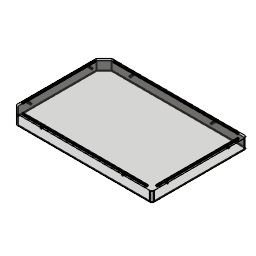
Design_2_Assembly (Autodesk Fusion 360 archive; units mm, degrees)
design "GREINER 96 WELL PLATE LID"
part number: 2026-02-05-10-27-23-618
Autodesk Fusion 360 part; units mm, degrees
sketch "Sketch1" plane through (0, 0, 0) normal (0, 0, 1) x (1, 0, 0)
  line L0 (61.42, -42.3) -> (-56.55, -42.3)
  line L1 (-63.55, -35.3) -> (-63.55, 35.3)
  line L2 (-56.55, 42.3) -> (61.42, 42.3)
  line L3 (63.55, 40.17) -> (63.55, -40.17)
  line L4 (63.55, -42.3) -> (-63.55, 42.3) construction
  line L5 (-63.55, -42.3) -> (63.55, 42.3) construction
  line L6 (-56.55, 42.3) -> (-63.55, 35.3)
  line L7 (0, -42.3) -> (0, 42.3) construction
  line L8 (63.55, 0) -> (-63.55, 0) construction
  line L9 (-56.55, -42.3) -> (-63.55, -35.3)
  arc A0 (63.55, 40.17) -> (61.42, 42.3) centre (61.42, 40.17) ccw
  arc A1 (61.42, -42.3) -> (63.55, -40.17) centre (61.42, -40.17) ccw
  dimension "d1" = 84.6
  dimension "d2" = 127.1
  dimension "d3" = 7
  dimension "d4" = 7
  dimension "d5" = 2.13
  constraint horizontal L0
  constraint perpendicular L0 L1
  constraint parallel L0 L2
  constraint parallel L1 L3
  constraint coincident L4 origin
  constraint coincident L5 origin
  constraint coincident L4.end L2
  constraint coincident L4.end L1
  constraint coincident L2 L7.end
  constraint perpendicular L2 L7
  constraint coincident L1 L8.end
  constraint perpendicular L1 L8
  constraint symmetric L2.start L8 L0.end
  constraint symmetric L1.end L8 L1.start
  constraint coincident L0 L7.start
  constraint coincident L3 L8.start
  constraint coincident L5.end L2
  constraint coincident L5.end L3
  constraint tangent L2 A0
  constraint tangent L3 A0
  constraint symmetric L8 L2.end L0.start
  constraint symmetric L8 L3.start L3.end
  constraint symmetric L8 A0 A1
  measures "d1" distance of L5.start L4.end
  measures "d2" distance of L4.end L5.end
  measures "d3" distance of L4.end L2.start
  measures "d4" distance of L4.end L1.end
  measures "d5" radius of A0
extrude "Extrude1" add sketch "Sketch1" against normal blind 9
sketch "Sketch2" plane through (0, 0, -9) normal (0, 0, -1) x (1, 0, 0)
  line L0 (61.42, 42.3) -> (-56.55, 42.3)
  line L1 (-56.55, 42.3) -> (-63.55, 35.3)
  line L2 (-63.55, 35.3) -> (-63.55, -35.3)
  line L3 (-63.55, -35.3) -> (-56.55, -42.3)
  line L4 (-56.55, -42.3) -> (61.42, -42.3)
  arc A0 (61.42, -42.3) -> (63.55, -40.17) centre (61.42, -40.17) ccw
  line L5 (63.55, -40.17) -> (63.55, 40.17)
  arc A1 (63.55, 40.17) -> (61.42, 42.3) centre (61.42, 40.17) ccw
  line L6 (61.42, -41.3) -> (-56.1358, -41.3)
  line L7 (-62.55, -34.8858) -> (-62.55, 34.8858)
  line L8 (-56.1358, 41.3) -> (61.42, 41.3)
  line L9 (62.55, 40.17) -> (62.55, -40.17)
  line L10 (62.55, -41.3) -> (-62.55, 41.3) construction
  line L11 (-62.55, -41.3) -> (62.55, 41.3) construction
  line L12 (-56.1358, 41.3) -> (-62.55, 34.8858)
  arc A2 (62.55, 40.17) -> (61.42, 41.3) centre (61.42, 40.17) ccw
  line L13 (63.55, 0) -> (-63.55, 0) construction
  line L14 (-56.1358, -41.3) -> (-62.55, -34.8858)
  arc A3 (61.42, -41.3) -> (62.55, -40.17) centre (61.42, -40.17) ccw
  dimension "d8" = 125.1
  dimension "d9" = 82.6
  dimension "d10" = 6.4142
  dimension "d11" = 6.4142
  dimension "d12" = 1
  dimension "d13" = 1.13
  constraint horizontal L6
  constraint perpendicular L6 L7
  constraint parallel L6 L8
  constraint parallel L7 L9
  constraint coincident L10 origin
  constraint coincident L11 origin
  constraint coincident L10.end L8
  constraint coincident L10.end L7
  constraint coincident L11.end L9
  constraint coincident L11.end L8
  constraint tangent L9 A2
  constraint tangent L8 A2
  constraint midpoint L5 L13.start
  constraint midpoint L2 L13.end
  constraint symmetric L8.start L13 L6.end
  constraint symmetric L7.end L13 L7.start
  constraint symmetric L9.start L13 L9.end
  constraint symmetric L8.end L13 L6.start
  constraint symmetric A2 L13 A3
  measures "d8" distance of L10.end L11.end
  measures "d9" distance of L11.start L10.end
  measures "d10" distance of L10.end L8.start
  measures "d11" distance of L10.end L7.end
  measures "d12" distance of L1 L12
  measures "d13" radius of A2
extrude "Extrude2" cut sketch "Sketch2" against normal blind 8 contours L6 L7 L8 L9 L12 A2 L14 A3
sketch "Sketch3" plane through (0, 0, -1) normal (0, 0, -1) x (1, 0, 0)
  line L0 (-56.1358, -41.3) -> (61.42, -41.3)
  arc A0 (61.42, -41.3) -> (62.55, -40.17) centre (61.42, -40.17) ccw
  line L1 (62.55, -40.17) -> (62.55, 40.17)
  arc A1 (62.55, 40.17) -> (61.42, 41.3) centre (61.42, 40.17) ccw
  line L2 (61.42, 41.3) -> (-56.1358, 41.3)
  line L3 (-56.1358, 41.3) -> (-62.55, 34.8858)
  line L4 (-62.55, 34.8858) -> (-62.55, -34.8858)
  line L5 (-62.55, -34.8858) -> (-56.1358, -41.3)
  line L6 (-62.55, 32.8642) -> (-35.55, 32.8642) construction
  line L7 (-35.55, 32.8642) -> (-35.55, 41.3) construction
  line L8 (-35.55, 41.3) -> (-36.55, 41.3)
  line L9 (-36.55, 41.3) -> (-36.55, 37.5)
  line L10 (-36.55, 37.5) -> (-35.55, 37.5)
  line L11 (-35.55, 37.5) -> (-35.55, 41.3)
  line L12 (-50.2731, 41.3) -> (-50.2731, 26.6) construction
  line L13 (-50.2731, 26.6) -> (-62.55, 26.6) construction
  line L14 (-62.55, 26.6) -> (-58.75, 26.6)
  line L15 (-58.75, 26.6) -> (-58.75, 27.6)
  line L16 (-58.75, 27.6) -> (-62.55, 27.6)
  line L17 (-62.55, 27.6) -> (-62.55, 26.6)
  line L18 (62.55, 0) -> (-62.55, 0) construction
  line L19 (-62.55, 30.673) -> (-62.55, 55) construction
  line L20 (62.55, 34.8173) -> (62.55, 55) construction
  line L21 (62.55, 55) -> (-62.55, 55) construction
  line L22 (0, 55) -> (0, -41.3) construction
  line L23 (62.55, 27.6) -> (62.55, 26.6)
  line L24 (62.55, 26.6) -> (58.75, 26.6)
  line L25 (58.75, 27.6) -> (62.55, 27.6)
  line L26 (58.75, 26.6) -> (58.75, 27.6)
  line L27 (36.55, 41.3) -> (36.55, 37.5)
  line L28 (35.55, 37.5) -> (35.55, 41.3)
  line L29 (36.55, 37.5) -> (35.55, 37.5)
  line L30 (35.55, 41.3) -> (36.55, 41.3)
  line L31 (62.55, -26.6) -> (58.75, -26.6)
  line L32 (58.75, -27.6) -> (62.55, -27.6)
  line L33 (58.75, -26.6) -> (58.75, -27.6)
  line L34 (35.55, -37.5) -> (35.55, -41.3)
  line L35 (36.55, -37.5) -> (35.55, -37.5)
  line L36 (36.55, -41.3) -> (36.55, -37.5)
  line L37 (62.55, -27.6) -> (62.55, -26.6)
  line L38 (35.55, -41.3) -> (36.55, -41.3)
  line L39 (-58.75, -26.6) -> (-58.75, -27.6)
  line L40 (-62.55, -26.6) -> (-58.75, -26.6)
  line L41 (-58.75, -27.6) -> (-62.55, -27.6)
  line L42 (-62.55, -27.6) -> (-62.55, -26.6)
  line L43 (-36.55, -37.5) -> (-35.55, -37.5)
  line L44 (-35.55, -37.5) -> (-35.55, -41.3)
  line L45 (-36.55, -41.3) -> (-36.55, -37.5)
  line L46 (-35.55, -41.3) -> (-36.55, -41.3)
  dimension "d16" = 27
  dimension "d17" = 3.8
  dimension "d18" = 1
  dimension "d19" = 14.7
  dimension "d20" = 3.8
  dimension "d21" = 1
  constraint coincident L4 L6.start
  constraint perpendicular L4 L6
  constraint coincident L2 L7.end
  constraint perpendicular L2 L7
  constraint horizontal L8
  constraint vertical L9
  constraint horizontal L10
  constraint vertical L11
  constraint coincident L2 L12.start
  constraint perpendicular L2 L12
  constraint coincident L4 L13.end
  constraint perpendicular L4 L13
  constraint horizontal L14
  constraint vertical L15
  constraint horizontal L16
  constraint vertical L17
  constraint midpoint L1 L18.start
  constraint midpoint L4 L18.end
  constraint coincident L4 L19.start
  constraint perpendicular L6 L19
  constraint coincident L1 L20.start
  constraint parallel L1 L20
  constraint perpendicular L19 L21
  constraint midpoint L21 L22.start
  constraint coincident L0 L22.end
  constraint perpendicular L0 L22
  constraint symmetric L7.end L22 L28.end
  constraint symmetric L8.end L22 L27.start
  constraint symmetric L9.end L22 L27.end
  constraint symmetric L10.end L22 L28.start
  constraint symmetric L13.end L22 L23.end
  constraint symmetric L14.end L22 L24.end
  constraint symmetric L15.end L22 L25.start
  constraint symmetric L16.end L22 L23.start
  constraint symmetric L7.end L18 L44.end
  constraint symmetric L8.end L18 L45.start
  constraint symmetric L9.end L18 L43.start
  constraint symmetric L10.end L18 L43.end
  constraint symmetric L13.end L18 L40.start
  constraint symmetric L14.end L18 L39.start
  constraint symmetric L15.end L18 L39.end
  constraint symmetric L16.end L18 L41.end
  constraint symmetric L18 L23.start L32.end
  constraint symmetric L18 L23.end L31.start
  constraint symmetric L18 L27.end L35.start
  constraint symmetric L18 L28.start L34.start
  constraint symmetric L18 L24.end L31.end
  constraint symmetric L18 L25.start L32.start
  constraint symmetric L18 L27.start L36.start
  constraint symmetric L18 L28.end L34.end
  measures "d16" distance of L6.start L6.end
  measures "d17" distance of L8.end L9.end
  measures "d18" distance of L9.end L10.end
  measures "d19" distance of L12.start L12.end
  measures "d20" distance of L15.end L16.end
  measures "d21" distance of L14.end L15.end
extrude "Extrude3" add sketch "Sketch3" along normal blind 1 contours L0 L43 L44 L45 L46 | L4 L39 L40 L41 L42 | L0 L34 L35 L36 L38 | L4 L14 L15 L16 L17 | L1 L31 L32 L33 L37 | L2 L8 L9 L10 L11 | L1 L23 L24 L25 L26 | L2 L27 L28 L29 L30
sketch "Sketch4" plane through (0, 0, 0) normal (0, 0, 1) x (-1, 0, 0)
  line L0 (56.55, 42.3) -> (-61.42, 42.3)
  arc A0 (-61.42, 42.3) -> (-63.55, 40.17) centre (-61.42, 40.17) ccw
  line L1 (-63.55, 40.17) -> (-63.55, -40.17)
  arc A1 (-63.55, -40.17) -> (-61.42, -42.3) centre (-61.42, -40.17) ccw
  line L2 (-61.42, -42.3) -> (56.55, -42.3)
  line L3 (56.55, -42.3) -> (63.55, -35.3)
  line L4 (63.55, -35.3) -> (63.55, 35.3)
  line L5 (63.55, 35.3) -> (56.55, 42.3)
  line L6 (-63.55, -34.3916) -> (-62.25, -34.3916) construction
  line L7 (-62.25, -34.3916) -> (-62.25, -36.4) construction
  line L8 (-60, -42.3) -> (-66.2, -42.3) construction
  line L9 (-63.55, -39.2433) -> (-63.55, -43.1) construction
  line L10 (-62.25, -36.4) -> (-60.95, -36.4)
  line L11 (-60.95, -36.4) -> (-60.95, 36.4)
  line L12 (-60.95, 36.4) -> (-62.25, 36.4)
  line L13 (-62.25, 36.4) -> (-62.25, -36.4)
  line L14 (-52.6219, -42.3) -> (-52.6219, -41) construction
  line L15 (-52.6219, -41) -> (-57.65, -41) construction
  line L16 (-57.65, -41) -> (53.05, -41)
  line L17 (53.05, -41) -> (53.05, -39.7)
  line L18 (53.05, -39.7) -> (-57.65, -39.7)
  line L19 (-57.65, -39.7) -> (-57.65, -41)
  line L20 (53.05, 39.7) -> (-57.65, 39.7)
  line L21 (-57.65, 41) -> (53.05, 41)
  line L22 (-57.65, 39.7) -> (-57.65, 41)
  line L23 (53.05, 41) -> (53.05, 39.7)
  line L24 (60.95, 0) -> (60.95, -32.3)
  line L25 (60.95, -32.3) -> (62.25, -32.3)
  line L26 (62.25, -32.3) -> (62.25, 0)
  line L27 (60.95, 0) -> (60.95, 32.3)
  line L28 (62.25, 32.3) -> (62.25, 0)
  line L29 (60.95, 32.3) -> (62.25, 32.3)
  line L30 (-63.55, 0) -> (60.95, 0) construction
  line L31 (62.25, 0) -> (63.55, 0) construction
  dimension "d24" = 1.3
  dimension "d25" = 5.9
  dimension "d26" = 72.8
  dimension "d27" = 1.3
  dimension "d28" = 1.3
  dimension "d29" = 5.9
  dimension "d30" = 1.3
  dimension "d31" = 110.7
  dimension "d32" = 32.3
  dimension "d33" = 1.3
  dimension "d34" = 1.3
  constraint coincident L1 L6.start
  constraint perpendicular L1 L6
  constraint perpendicular L6 L7
  constraint coincident L2 L8.start
  constraint parallel L2 L8
  constraint coincident L1 L9.start
  constraint perpendicular L2 L9
  constraint horizontal L10
  constraint vertical L11
  constraint horizontal L12
  constraint vertical L13
  constraint coincident L2 L14.start
  constraint perpendicular L2 L14
  constraint perpendicular L14 L15
  constraint horizontal L16
  constraint vertical L17
  constraint horizontal L18
  constraint vertical L19
  constraint midpoint L1 L30.start
  constraint midpoint L4 L31.end
  constraint symmetric L15.end L21.start L30
  constraint symmetric L16.end L21.end L30
  constraint symmetric L17.end L20.start L30
  constraint symmetric L18.end L20.end L30
  constraint vertical L24
  constraint horizontal L25
  constraint vertical L26
  constraint symmetric L24.end L27.end L30
  constraint symmetric L25.end L28.start L31
  constraint collinear L30 L31
  measures "d24" distance of L6.start L6.end
  measures "d25" distance of L7.end L8
  measures "d26" distance of L10.end L11.end
  measures "d27" distance of L7.end L10.end
  measures "d28" distance of L14.start L14.end
  measures "d29" distance of L9 L15.end
  measures "d30" distance of L15.end L18.end
  measures "d31" distance of L17.end L18.end
  measures "d32" distance of L24.start L24.end
  measures "d33" distance of L24.end L25.end
  measures "d34" distance of L4 L26
extrude "Extrude4" add sketch "Sketch4" along normal blind 1 contours L10 L11 L12 L13 | L16 L17 L18 L19 | L20 L21 L22 L23 | L24 L25 L26 L27 L28 L29
equation "d4 = d3"
equation "d11 = d10"

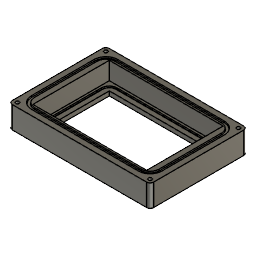
design "Base V2.1"
part number: 2026-01-30-14-30-51-369
Autodesk Fusion 360 part; units mm, degrees
sketch "Sketch1" plane through (0, 0, 0) normal (0, 0, 1) x (1, 0, 0)
  line L0 (76, -55) -> (-76, -55)
  line L1 (-80, -51) -> (-80, 51)
  line L2 (-76, 55) -> (76, 55)
  line L3 (80, 51) -> (80, -51)
  line L4 (80, -55) -> (-80, 55) construction
  line L5 (-80, -55) -> (80, 55) construction
  arc A0 (-76, 55) -> (-80, 51) centre (-76, 51) ccw
  arc A1 (80, 51) -> (76, 55) centre (76, 51) ccw
  arc A2 (76, -55) -> (80, -51) centre (76, -51) ccw
  arc A3 (-80, -51) -> (-76, -55) centre (-76, -51) ccw
  circle A4 centre (-75, 50) radius 2
  line L6 (0, 55) -> (0, -55) construction
  line L7 (80, 0) -> (-80, 0) construction
  circle A5 centre (75, 50) radius 2
  circle A6 centre (75, -50) radius 2
  circle A7 centre (-75, -50) radius 2
  dimension "d1" = 160
  dimension "d2" = 110
  dimension "d26" = 4
  dimension "d27" = 4
  dimension "d28" = 4
  dimension "d29" = 4
  dimension "d30" = 4
  dimension "d31" = 5
  dimension "d32" = 5
  constraint horizontal L0
  constraint perpendicular L0 L1
  constraint parallel L0 L2
  constraint parallel L1 L3
  constraint coincident L4 origin
  constraint coincident L5 origin
  constraint coincident L4.end L2
  constraint coincident L4.end L1
  constraint tangent L2 A0
  constraint tangent L1 A0
  constraint coincident L5.end L3
  constraint coincident L5.end L2
  constraint tangent L3 A1
  constraint tangent L2 A1
  constraint coincident L4.start L3
  constraint coincident L4.start L0
  constraint tangent L3 A2
  constraint tangent L0 A2
  constraint coincident L5.start L1
  constraint coincident L5.start L0
  constraint tangent L1 A3
  constraint tangent L0 A3
  constraint midpoint L2 L6.start
  constraint midpoint L0 L6.end
  constraint midpoint L3 L7.start
  constraint midpoint L1 L7.end
  constraint symmetric A4 L6 A5
  constraint symmetric A4 L7 A7
  constraint symmetric L7 A5 A6
  measures "d1" distance of L4.end L5.end
  measures "d2" distance of L5.start L4.end
  measures "d26" radius of A0
  measures "d27" radius of A1
  measures "d28" radius of A2
  measures "d29" radius of A3
  measures "d30" diameter of A4
  measures "d31" distance of L2 A4.centre
  measures "d32" distance of L1 A4.centre
extrude "Extrude1" add sketch "Sketch1" along normal blind 25
sketch "Sketch2" plane through (0, 0, 25) normal (0, 0, 1) x (-1, 0, 0)
  line L0 (-76, -55) -> (76, -55)
  line L1 (80, -51) -> (80, 51)
  line L2 (76, 55) -> (-76, 55)
  line L3 (-80, 51) -> (-80, -51)
  line L4 (-64.4, 43.25) -> (64.4, 43.25)
  line L5 (64.4, 43.25) -> (64.4, -43.25)
  line L6 (64.4, -43.25) -> (-64.4, -43.25)
  line L7 (-64.4, -43.25) -> (-64.4, 43.25)
  line L8 (-64.4, 43.25) -> (64.4, -43.25) construction
  line L9 (64.4, 43.25) -> (-64.4, -43.25) construction
  arc A0 (76, -55) -> (80, -51) centre (76, -51) ccw
  arc A1 (80, 51) -> (76, 55) centre (76, 51) ccw
  arc A2 (-76, 55) -> (-80, 51) centre (-76, 51) ccw
  arc A3 (-80, -51) -> (-76, -55) centre (-76, -51) ccw
  circle A4 centre (75, 50) radius 2
  circle A5 centre (-75, 50) radius 2
  circle A6 centre (-75, -50) radius 2
  circle A7 centre (75, -50) radius 2
  dimension "d5" = 128.8
  dimension "d6" = 86.5
  constraint horizontal L4
  constraint perpendicular L4 L5
  constraint parallel L4 L6
  constraint parallel L5 L7
  constraint coincident L8 origin
  constraint coincident L9 origin
  measures "d5" distance of L5.end L6.end
  measures "d6" distance of L4.end L5.end
extrude "Extrude2" cut sketch "Sketch2" against normal blind 20 contours L4 L5 L6 L7
sketch "Sketch3" plane through (0, 0, 25) normal (0, 0, 1) x (-1, 0, 0)
  line L0 (64.4, 43.25) -> (64.4, -43.25)
  line L1 (64.4, -43.25) -> (-64.4, -43.25)
  line L2 (-64.4, -43.25) -> (-64.4, 43.25)
  line L3 (-64.4, 43.25) -> (64.4, 43.25)
  line L4 (-76, -55) -> (76, -55)
  line L5 (80, -51) -> (80, 51)
  line L6 (76, 55) -> (-76, 55)
  line L7 (-80, 51) -> (-80, -51)
  line L8 (-72.0964, 47.0964) -> (72.0964, 47.0964) construction
  line L9 (72.0964, 47.0964) -> (72.0964, -47.0964) construction
  line L10 (72.0964, -47.0964) -> (-72.0964, -47.0964) construction
  line L11 (-72.0964, -47.0964) -> (-72.0964, 47.0964) construction
  line L12 (-72.0964, 47.0964) -> (72.0964, -47.0964) construction
  line L13 (72.0964, 47.0964) -> (-72.0964, -47.0964) construction
  line L14 (70.6619, 35.3929) -> (70.6619, -35.3929)
  line L15 (60.3929, -45.6619) -> (-60.3929, -45.6619)
  line L16 (-70.6619, -35.3929) -> (-70.6619, 35.3929)
  line L17 (-70.6619, 45.6619) -> (70.6619, -45.6619) construction
  line L18 (70.6619, 45.6619) -> (-70.6619, -45.6619) construction
  line L19 (-60.3929, 48.5309) -> (60.3929, 48.5309)
  line L20 (73.5309, 35.3929) -> (73.5309, -35.3929)
  line L21 (60.3929, -48.5309) -> (-60.3929, -48.5309)
  line L22 (-73.5309, -35.3929) -> (-73.5309, 35.3929)
  line L23 (-73.5309, 48.5309) -> (73.5309, -48.5309) construction
  line L24 (73.5309, 48.5309) -> (-73.5309, -48.5309) construction
  arc A0 (60.3929, -45.6619) -> (70.6619, -35.3929) centre (60.3929, -35.3929) ccw
  arc A1 (60.3929, -48.5309) -> (73.5309, -35.3929) centre (60.3929, -35.3929) ccw
  line L25 (0, -55) -> (0, 55) construction
  line L26 (-80, 0) -> (80, 0) construction
  arc A2 (-70.6619, -35.3929) -> (-60.3929, -45.6619) centre (-60.3929, -35.3929) ccw
  arc A3 (-73.5309, -35.3929) -> (-60.3929, -48.5309) centre (-60.3929, -35.3929) ccw
  arc A4 (-60.3929, 45.6619) -> (-70.6619, 35.3929) centre (-60.3929, 35.3929) ccw
  arc A5 (-60.3929, 48.5309) -> (-73.5309, 35.3929) centre (-60.3929, 35.3929) ccw
  arc A6 (70.6619, 35.3929) -> (60.3929, 45.6619) centre (60.3929, 35.3929) ccw
  arc A7 (73.5309, 35.3929) -> (60.3929, 48.5309) centre (60.3929, 35.3929) ccw
  line L27 (-60.3929, 45.6619) -> (60.3929, 45.6619)
  arc A8 (76, -55) -> (80, -51) centre (76, -51) ccw
  arc A9 (80, 51) -> (76, 55) centre (76, 51) ccw
  arc A10 (-76, 55) -> (-80, 51) centre (-76, 51) ccw
  arc A11 (-80, -51) -> (-76, -55) centre (-76, -51) ccw
  circle A12 centre (75, 50) radius 2
  circle A13 centre (-75, 50) radius 2
  circle A14 centre (-75, -50) radius 2
  circle A15 centre (75, -50) radius 2
  dimension "d9" = 144.1928
  dimension "d15" = 94.1928
  dimension "d16" = 1.4345
  dimension "d17" = 1.4345
  dimension "d18" = 1.4345
  dimension "d19" = 1.4345
  dimension "d20" = 10.269
  dimension "d21" = 13.138
  constraint horizontal L8
  constraint perpendicular L8 L9
  constraint parallel L8 L10
  constraint parallel L9 L11
  constraint coincident L12 origin
  constraint coincident L13 origin
  constraint parallel L15 L27
  constraint parallel L14 L16
  constraint coincident L17 origin
  constraint coincident L18 origin
  constraint horizontal L19
  constraint perpendicular L19 L20
  constraint parallel L19 L21
  constraint parallel L20 L22
  constraint coincident L23 origin
  constraint coincident L24 origin
  constraint coincident L17.end L15
  constraint coincident L17.end L14
  constraint tangent L15 A0
  constraint tangent L14 A0
  constraint coincident L23.end L21
  constraint coincident L23.end L20
  constraint tangent L21 A1
  constraint tangent L20 A1
  constraint midpoint L4 L25.start
  constraint midpoint L6 L25.end
  constraint midpoint L7 L26.start
  constraint midpoint L5 L26.end
  constraint symmetric L15.start L25 L15.end
  constraint symmetric L14.end L25 L16.start
  constraint symmetric A0 L25 A2
  constraint symmetric L21.start L25 L21.end
  constraint symmetric L20.end L25 L22.start
  constraint symmetric A1 L25 A3
  constraint symmetric L15.start L26 A6.end
  constraint symmetric L14.end L26 L14.start
  constraint symmetric A0 L26 A6
  constraint symmetric L21.start L26 L19.end
  constraint symmetric L20.end L26 L20.start
  constraint symmetric A1 L26 A7
  constraint symmetric L26 L15.end A4.start
  constraint symmetric L26 L16.start L16.end
  constraint symmetric L26 A2 A4
  constraint symmetric L26 L21.end L19.start
  constraint symmetric L26 L22.start L22.end
  constraint symmetric L26 A3 A5
  measures "d9" distance of L8.start L8.end
  measures "d15" distance of L8 L10
  measures "d16" distance of L11 L16
  measures "d17" distance of L10 L15
  measures "d18" distance of L11 L22
  measures "d19" distance of L10 L21
  measures "d20" radius of A0
  measures "d21" radius of A1
extrude "Extrude3" cut sketch "Sketch3" against normal blind 1.424 contours L19 L20 L21 L22 A1 A3 A5 A7
draft "Draft1" angle 10 neutral plane through (0, 0, 23.576) pull (0, 0, 1) 16 faces at (-70.6619, -11.7976, 24.5253) (-67.8249, 42.4793, 24.0507) (-20.131, 45.6619, 24.5253) (67.4793, 42.8249, 24.0507) (70.6619, 11.7976, 24.5253) (67.8249, -42.4793, 24.0507) (20.131, -45.6619, 24.5253) (-64.2095, -44.9263, 24.5253) (-73.5309, -11.7976, 24.5253) (-70.7201, -43.5143, 24.0507) (20.131, -48.5309, 24.5253) (68.5143, -45.7201, 24.0507) (73.5309, 11.7976, 24.5253) (70.7201, 43.5143, 24.0507) (-20.131, 48.5309, 24.5253) (-71.0948, 43.0137, 24.0507)
sketch "Sketch4" plane through (0, 0, 5) normal (0, 0, 1) x (-1, 0, 0)
  line L0 (-64.4, -43.25) -> (64.4, -43.25)
  line L1 (64.4, -43.25) -> (64.4, 43.25)
  line L2 (64.4, 43.25) -> (-64.4, 43.25)
  line L3 (-64.4, 43.25) -> (-64.4, -43.25)
  line L4 (-54.4, 33.25) -> (54.4, 33.25)
  line L5 (54.4, 33.25) -> (54.4, -33.25)
  line L6 (54.4, -33.25) -> (-54.4, -33.25)
  line L7 (-54.4, -33.25) -> (-54.4, 33.25)
  line L8 (-54.4, 33.25) -> (54.4, -33.25) construction
  line L9 (54.4, 33.25) -> (-54.4, -33.25) construction
  dimension "d35" = 10
  dimension "d36" = 10
  constraint horizontal L4
  constraint perpendicular L4 L5
  constraint parallel L4 L6
  constraint parallel L5 L7
  constraint coincident L8 origin
  constraint coincident L9 origin
  measures "d35" distance of L3 L7
  measures "d36" distance of L0 L6
extrude "Extrude4" cut sketch "Sketch4" against normal blind 5 contours L4 L5 L6 L7
sketch "Sketch5" plane through (0, 0, 5) normal (0, 0, 1) x (-1, 0, 0)
  line L0 (54.4, 33.25) -> (54.4, -33.25)
  line L1 (54.4, -33.25) -> (-54.4, -33.25)
  line L2 (-54.4, -33.25) -> (-54.4, 33.25)
  line L3 (-54.4, 33.25) -> (54.4, 33.25)
  line L4 (-64.4, -43.25) -> (64.4, -43.25)
  line L5 (64.4, -43.25) -> (64.4, 43.25)
  line L6 (64.4, 43.25) -> (-64.4, 43.25)
  line L7 (-64.4, 43.25) -> (-64.4, -43.25)
  line L8 (-60.8342, 39.6842) -> (60.8342, 39.6842) construction
  line L9 (60.8342, 39.6842) -> (60.8342, -39.6842) construction
  line L10 (60.8342, -39.6842) -> (-60.8342, -39.6842) construction
  line L11 (-60.8342, -39.6842) -> (-60.8342, 39.6842) construction
  line L12 (-60.8342, 39.6842) -> (60.8342, -39.6842) construction
  line L13 (60.8342, 39.6842) -> (-60.8342, -39.6842) construction
  line L14 (59.7842, 31.4252) -> (59.7842, -31.4252)
  line L15 (52.5752, -38.6342) -> (-52.5752, -38.6342)
  line L16 (-59.7842, -31.4252) -> (-59.7842, 31.4252)
  line L17 (-57.1085, 36.9051) -> (59.7842, -38.6342) construction
  line L18 (57.4574, 36.3074) -> (-57.4574, -36.3074) construction
  line L19 (-52.8062, 40.6187) -> (52.8062, 40.6187)
  line L20 (61.8842, 31.5407) -> (61.8842, -31.5407)
  line L21 (52.8062, -40.6187) -> (-52.8062, -40.6187)
  line L22 (-61.8842, -31.5407) -> (-61.8842, 31.5407)
  line L23 (-58.9962, 38.7231) -> (61.8842, -40.6187) construction
  line L24 (59.3264, 38.1764) -> (-59.3264, -38.1764) construction
  arc A0 (52.5752, -38.6342) -> (59.7842, -31.4252) centre (52.5752, -31.4252) ccw
  arc A1 (52.8062, -40.6187) -> (61.8842, -31.5407) centre (52.8062, -31.5407) ccw
  line L25 (0, -43.25) -> (0, 43.25) construction
  line L26 (-64.4, 0) -> (64.4, 0) construction
  arc A2 (-59.7842, -31.4252) -> (-52.5752, -38.6342) centre (-52.5752, -31.4252) ccw
  arc A3 (-61.8842, -31.5407) -> (-52.8062, -40.6187) centre (-52.8062, -31.5407) ccw
  arc A4 (59.7842, 31.4252) -> (52.5752, 38.6342) centre (52.5752, 31.4252) ccw
  arc A5 (61.8842, 31.5407) -> (52.8062, 40.6187) centre (52.8062, 31.5407) ccw
  arc A6 (-52.5752, 38.6342) -> (-59.7842, 31.4252) centre (-52.5752, 31.4252) ccw
  arc A7 (-52.8062, 40.6187) -> (-61.8842, 31.5407) centre (-52.8062, 31.5407) ccw
  line L27 (-52.5752, 38.6342) -> (52.5752, 38.6342)
  dimension "d42" = 121.6684
  dimension "d43" = 79.3684
  dimension "d44" = 1.05
  dimension "d45" = 0.9345
  dimension "d46" = 1.05
  dimension "d47" = 1.05
  dimension "d48" = 7.209
  dimension "d49" = 9.078
  constraint horizontal L8
  constraint perpendicular L8 L9
  constraint parallel L8 L10
  constraint parallel L9 L11
  constraint coincident L12 origin
  constraint coincident L13 origin
  constraint parallel L15 L27
  constraint parallel L14 L16
  constraint coincident L17 origin
  constraint coincident L18 origin
  constraint horizontal L19
  constraint perpendicular L19 L20
  constraint parallel L19 L21
  constraint parallel L20 L22
  constraint coincident L23 origin
  constraint coincident L24 origin
  constraint coincident L17.end L15
  constraint coincident L17.end L14
  constraint tangent L15 A0
  constraint tangent L14 A0
  constraint coincident L23.end L21
  constraint coincident L23.end L20
  constraint tangent L21 A1
  constraint tangent L20 A1
  constraint midpoint L4 L25.start
  constraint midpoint L6 L25.end
  constraint midpoint L7 L26.start
  constraint midpoint L5 L26.end
  constraint symmetric L15.start L25 L15.end
  constraint symmetric L14.end L25 L16.start
  constraint symmetric A0 L25 A2
  constraint symmetric L21.start L25 L21.end
  constraint symmetric L20.end L25 L22.start
  constraint symmetric A1 L25 A3
  constraint symmetric L15.start L26 A4.end
  constraint symmetric L14.end L26 L14.start
  constraint symmetric A0 L26 A4
  constraint symmetric L21.start L26 L19.end
  constraint symmetric L20.end L26 L20.start
  constraint symmetric A1 L26 A5
  constraint symmetric L26 L15.end A6.start
  constraint symmetric L26 L16.start L16.end
  constraint symmetric L26 A2 A6
  constraint symmetric L26 L21.end L19.start
  constraint symmetric L26 L22.start L22.end
  constraint symmetric L26 A3 A7
  measures "d42" distance of L9 L11
  measures "d43" distance of L8 L10
  measures "d44" distance of L11 L22
  measures "d45" distance of L8 L19
  measures "d46" distance of L8 L27
  measures "d47" distance of L11 L16
  measures "d48" radius of A0
  measures "d49" radius of A1
extrude "Extrude5" cut sketch "Sketch5" against normal blind 1.6 contours L19 L20 L21 L22 A1 A3 A5 A7
equation "d9 = ( ORingPerimeter - 100 mm ) / 4 + 50 mm"
equation "ORingDiameter = 1.78 mm" comment "Diamter of the O ring"
equation "ORingInnerDiameter = 150 mm" comment "Inner diamter of the o ring bore"
equation "ORingPerimeter = 2 * 3.1412 * ( ( ORingInnerDiameter / 2 ) + ORingDiameter / 2 )"
equation "PanelWidth = 80 mm"
equation "PanelLength = 115 mm"
equation "d15 = ( ORingPerimeter - 100 mm ) / 4"
equation "d16 = ( ( ORingDiameter * 1.05 ) / 2 ) + 0.5 mm"
equation "d17 = ( ( ORingDiameter * 1.05 ) / 2 ) + 0.5 mm"
equation "d18 = ( ( ORingDiameter * 1.05 ) / 2 ) + 0.5 mm"
equation "d19 = ( ( ORingDiameter * 1.05 ) / 2 ) + 0.5 mm"
equation "d20 = ( ORingDiameter ) * 6 + ORingDiameter * 0.05 - 0.5 mm"
equation "d21 = ( ORingDiameter ) * 6 + ( ORingDiameter * 1.1 ) + 0.5 mm"
equation "d22 = -ORingDiameter * 0.8"
equation "ORing2Diameter = 2 mm" comment "Second O ring Diameter"
equation "ORing2InnerDiameter = 126 mm" comment "Inner diameter of the second O Ring"
equation "ORing2Perimeter = 2 * 3.1412 * ( ( ORing2InnerDiameter / 2 ) + ORing2Diameter / 2 )"
equation "d42 = ( ORing2Perimeter - 84.6 mm ) / 4 + 42.3 mm"
equation "d43 = ( ORing2Perimeter - 84.6 mm ) / 4"
equation "d44 = ( ORing2Diameter * 1.05 ) / 2"
equation "d45 = ( ORingDiameter * 1.05 ) / 2"
equation "d46 = ( ORing2Diameter * 1.05 ) / 2"
equation "d47 = ( ORing2Diameter * 1.05 ) / 2"
equation "d48 = ( ORingDiameter ) * 4 + ORingDiameter * 0.05 - 0.0 mm"
equation "d49 = ( ORingDiameter ) * 4 + ORingDiameter * 1.1 + 0 mm"
equation "d50 = -ORing2Diameter * 0.8"

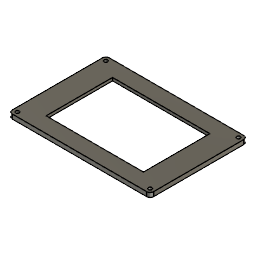
design "Lid V2 (O-Ring)"
part number: 2026-01-29-14-58-12-979
Autodesk Fusion 360 part; units mm, degrees
sketch "Sketch2" plane through (0, 0, 0) normal (0, 0, 1) x (1, 0, 0)
  line L0 (-46, 50) -> (106, 50)
  line L1 (110, 46) -> (110, -56)
  line L2 (106, -60) -> (-46, -60)
  line L3 (-50, -56) -> (-50, 46)
  circle A0 centre (-45, 45) radius 2
  line L4 (30, -60) -> (30, 50) construction
  line L5 (-50, -5) -> (110, -5) construction
  arc A1 (-46, 50) -> (-50, 46) centre (-46, 46) ccw
  circle A2 centre (105, 45) radius 2
  arc A3 (110, 46) -> (106, 50) centre (106, 46) ccw
  circle A4 centre (105, -55) radius 2
  arc A5 (106, -60) -> (110, -56) centre (106, -56) ccw
  circle A6 centre (-45, -55) radius 2
  arc A7 (-50, -56) -> (-46, -60) centre (-46, -56) ccw
  point P0 (-50, 50)
  point P1 (110, 50)
  dimension "d3" = 4
  dimension "d4" = 5
  dimension "d5" = 5
  dimension "d6" = 4
  dimension "d63" = 160
  dimension "d64" = 110
  constraint horizontal L0
  constraint vertical L1
  constraint horizontal L2
  constraint vertical L3
  constraint coincident L0 L4.end
  constraint coincident L3 L5.start
  constraint coincident P0 L0
  constraint coincident P0 L3
  constraint tangent L0 A1
  constraint tangent L3 A1
  constraint symmetric P0 L4 P1
  constraint symmetric A0 L4 A2
  constraint symmetric L4 L0.start L0.end
  constraint symmetric L4 L3.end L1.start
  constraint symmetric L4 A1 A3
  constraint coincident L1 L5.end
  constraint symmetric A0 L5 A6
  constraint symmetric L5 L0.start L2.end
  constraint symmetric L5 L3.end L3.start
  constraint symmetric L5 A1 A7
  constraint symmetric L5 L1.start L1.end
  constraint symmetric L5 L0.end L2.start
  constraint symmetric L5 A2 A4
  constraint symmetric L5 A3 A5
  constraint coincident L2 L4.start
  measures "d3" diameter of A0
  measures "d4" distance of L0 A0.centre
  measures "d5" distance of L3 A0.centre
  measures "d6" radius of A1
  measures "d63" distance of L1 L3
  measures "d64" distance of L0 L2
extrude "Extrude1" add sketch "Sketch2" along normal blind 5
sketch "Sketch3" plane through (0, 0, 0) normal (0, 0, -1) x (1, 0, 0)
  circle A0 centre (105, 55) radius 2
  circle A1 centre (-45, 55) radius 2
  circle A2 centre (-45, -45) radius 2
  circle A3 centre (105, -45) radius 2
  arc A4 (-50, -46) -> (-46, -50) centre (-46, -46) ccw
  line L0 (-46, -50) -> (106, -50)
  arc A5 (106, -50) -> (110, -46) centre (106, -46) ccw
  line L1 (110, -46) -> (110, 56)
  arc A6 (110, 56) -> (106, 60) centre (106, 56) ccw
  line L2 (106, 60) -> (-46, 60)
  arc A7 (-46, 60) -> (-50, 56) centre (-46, 56) ccw
  line L3 (-50, 56) -> (-50, -46)
  line L4 (30, 60) -> (30, -50) construction
  line L5 (110, 5) -> (-50, 5) construction
  line L6 (102.0964, -42.0964) -> (-42.0964, -42.0964) construction
  line L7 (-42.0964, -42.0964) -> (-42.0964, 52.0964) construction
  line L8 (-42.0964, 52.0964) -> (102.0964, 52.0964) construction
  line L9 (102.0964, 52.0964) -> (102.0964, -42.0964) construction
  line L10 (102.0964, -42.0964) -> (-42.0964, 52.0964) construction
  line L11 (-42.0964, -42.0964) -> (102.0964, 52.0964) construction
  line L12 (90.3929, -43.5309) -> (-30.3929, -43.5309)
  line L13 (-43.5309, -30.3929) -> (-43.5309, 40.3929)
  line L14 (-30.3929, 53.5309) -> (90.3929, 53.5309)
  line L15 (103.5309, 40.3929) -> (103.5309, -30.3929)
  line L16 (88.8372, -33.833) -> (-43.5309, 53.5309) construction
  line L17 (-37.4412, -35.28) -> (85.6746, 38.2522) construction
  line L18 (-40.6619, -30.3929) -> (-40.6619, 40.3929)
  line L19 (-30.3929, 50.6619) -> (90.3929, 50.6619)
  line L20 (100.6619, 40.3929) -> (100.6619, -30.3929)
  line L21 (98.0436, -38.97) -> (-40.6619, 50.6619) construction
  line L22 (-34.7613, -32.5014) -> (82.9436, 35.6581) construction
  arc A8 (-30.3929, 50.6619) -> (-40.6619, 40.3929) centre (-30.3929, 40.3929) ccw
  arc A9 (-30.3929, 53.5309) -> (-43.5309, 40.3929) centre (-30.3929, 40.3929) ccw
  arc A10 (100.6619, 40.3929) -> (90.3929, 50.6619) centre (90.3929, 40.3929) ccw
  arc A11 (103.5309, 40.3929) -> (90.3929, 53.5309) centre (90.3929, 40.3929) ccw
  arc A12 (-40.6619, -30.3929) -> (-30.3929, -40.6619) centre (-30.3929, -30.3929) ccw
  arc A13 (-43.5309, -30.3929) -> (-30.3929, -43.5309) centre (-30.3929, -30.3929) ccw
  arc A14 (90.3929, -40.6619) -> (100.6619, -30.3929) centre (90.3929, -30.3929) ccw
  arc A15 (90.3929, -43.5309) -> (103.5309, -30.3929) centre (90.3929, -30.3929) ccw
  line L23 (90.3929, -40.6619) -> (-30.3929, -40.6619)
  point P0 (30, 5)
  point P1 (30, 5)
  point P2 (30, 5)
  point P3 (30, 5)
  point P4 (30, 5)
  dimension "d25" = 144.1928
  dimension "d27" = 94.1928
  dimension "d28" = 1.4345
  dimension "d29" = 1.4345
  dimension "d30" = 1.4345
  dimension "d31" = 1.4345
  dimension "d44" = 10.269
  dimension "d45" = 13.138
  constraint midpoint L2 L4.start
  constraint midpoint L0 L4.end
  constraint midpoint L1 L5.start
  constraint midpoint L3 L5.end
  constraint midpoint L4 P4
  constraint coincident P4 P3
  constraint horizontal L6
  constraint perpendicular L6 L7
  constraint parallel L6 L8
  constraint parallel L7 L9
  constraint coincident L10 P4
  constraint coincident L11 P4
  constraint horizontal L12
  constraint perpendicular L12 L13
  constraint parallel L12 L14
  constraint parallel L13 L15
  constraint coincident L16 P4
  constraint coincident L17 P4
  constraint perpendicular L18 L23
  constraint parallel L19 L23
  constraint parallel L18 L20
  constraint coincident L21 P4
  constraint coincident L22 P4
  constraint coincident L21.end L19
  constraint coincident L21.end L18
  constraint tangent L19 A8
  constraint tangent L18 A8
  constraint coincident L16.end L14
  constraint coincident L16.end L13
  constraint tangent L14 A9
  constraint tangent L13 A9
  constraint symmetric L4 L19.start L19.end
  constraint symmetric L4 L18.end L20.start
  constraint symmetric L4 A8 A10
  constraint symmetric L4 L14.start L14.end
  constraint symmetric L4 L13.end L15.start
  constraint symmetric L4 A9 A11
  constraint symmetric L5 L19.start A12.end
  constraint symmetric L5 L18.end L18.start
  constraint symmetric L5 A8 A12
  constraint symmetric L5 L14.start L12.end
  constraint symmetric L5 L13.end L13.start
  constraint symmetric L5 A9 A13
  constraint symmetric L5 L19.end A14.start
  constraint symmetric L5 L20.start L20.end
  constraint symmetric L5 A10 A14
  constraint symmetric L5 L14.end L12.start
  constraint symmetric L5 L15.start L15.end
  constraint symmetric L5 A11 A15
  measures "d25" distance of L7.end L8.end
  measures "d27" distance of L6.end L7.end
  measures "d28" distance of L9 L15
  measures "d29" distance of L8 L14
  measures "d30" distance of L8 L19
  measures "d31" distance of L9 L20
  measures "d44" radius of A8
  measures "d45" radius of A9
extrude "Extrude4" add sketch "Sketch3" along normal blind 1.424 contours L12 L13 L14 L15 A9 A11 A13 A15
draft "Draft3" angle 10 neutral plane through (0, 0, -1.424) pull (0, 0, -1) 16 faces at (9.869, -50.6619, -0.9493) (96.3495, -48.7578, -0.9493) (100.6619, -16.7976, -0.4747) (92.8139, 40.3724, -0.9493) (9.869, 40.6619, -0.9493) (-33.7516, 40.0971, -0.9493) (-40.6619, 6.7976, -0.4747) (-40.0971, -43.7516, -0.9493) (-43.5309, 6.7976, -0.4747) (-38.0137, 41.0948, -0.9493) (50.131, 43.5309, -0.4747) (103.516, 31.018, -0.9493) (103.5309, -16.7976, -0.9493) (99.4592, -49.9013, -0.9493) (9.869, -53.5309, -0.4747) (-38.5143, -50.7201, -0.9493)
sketch "Sketch5" plane through (0, 0, -1.424) normal (0, 0, -1) x (1, 0, 0)
  line L0 (-30.3929, 50.6619) -> (90.3929, 50.6619)
  line L1 (100.6619, 40.3929) -> (100.6619, -30.3929)
  line L2 (90.3929, -40.6619) -> (-30.3929, -40.6619)
  line L3 (-40.6619, -30.3929) -> (-40.6619, 40.3929)
  line L4 (90.3929, 53.5309) -> (-30.3929, 53.5309)
  line L5 (-43.5309, 40.3929) -> (-43.5309, -30.3929)
  line L6 (-30.3929, -43.5309) -> (90.3929, -43.5309)
  line L7 (103.5309, -30.3929) -> (103.5309, 40.3929)
  line L8 (30, 53.5309) -> (30, -43.5309) construction
  line L9 (103.5309, 5) -> (-43.5309, 5) construction
  line L10 (102.0964, -42.0964) -> (-42.0964, -42.0964) construction
  line L11 (-42.0964, -42.0964) -> (-42.0964, 52.0964) construction
  line L12 (-42.0964, 52.0964) -> (102.0964, 52.0964) construction
  line L13 (102.0964, 52.0964) -> (102.0964, -42.0964) construction
  line L14 (102.0964, -42.0964) -> (-42.0964, 52.0964) construction
  line L15 (-42.0964, -42.0964) -> (102.0964, 52.0964) construction
  line L16 (90.3929, -43.0309) -> (-30.3929, -43.0309)
  line L17 (-43.0309, -30.3929) -> (-43.0309, 40.3929)
  line L18 (-30.3929, 53.0309) -> (90.3929, 53.0309)
  line L19 (103.0309, 40.3929) -> (103.0309, -30.3929)
  line L20 (88.9806, -33.7903) -> (-43.0309, 53.0309) construction
  line L21 (-43.0309, -43.0309) -> (88.9807, 43.7903) construction
  line L22 (90.3929, -41.1619) -> (-30.3929, -41.1619)
  line L23 (-41.1619, -30.3929) -> (-41.1619, 40.3929)
  line L24 (101.1619, 40.3929) -> (101.1619, -30.3929)
  line L25 (88.054, -32.659) -> (-41.1619, 51.1619) construction
  line L26 (-41.1619, -41.1619) -> (88.054, 42.659) construction
  arc A0 (100.6619, 40.3929) -> (90.3929, 50.6619) centre (90.3929, 40.3929) ccw
  arc A1 (90.3929, -40.6619) -> (100.6619, -30.3929) centre (90.3929, -30.3929) ccw
  arc A2 (-40.6619, -30.3929) -> (-30.3929, -40.6619) centre (-30.3929, -30.3929) ccw
  arc A3 (-30.3929, 50.6619) -> (-40.6619, 40.3929) centre (-30.3929, 40.3929) ccw
  arc A4 (-43.5309, -30.3929) -> (-30.3929, -43.5309) centre (-30.3929, -30.3929) ccw
  arc A5 (90.3929, -43.5309) -> (103.5309, -30.3929) centre (90.3929, -30.3929) ccw
  arc A6 (103.5309, 40.3929) -> (90.3929, 53.5309) centre (90.3929, 40.3929) ccw
  arc A7 (-30.3929, 53.5309) -> (-43.5309, 40.3929) centre (-30.3929, 40.3929) ccw
  arc A8 (-30.3929, 51.1619) -> (-41.1619, 40.3929) centre (-30.3929, 40.3929) ccw
  arc A9 (-30.3929, 53.0309) -> (-43.0309, 40.3929) centre (-30.3929, 40.3929) ccw
  arc A10 (101.1619, 40.3929) -> (90.3929, 51.1619) centre (90.3929, 40.3929) ccw
  arc A11 (103.0309, 40.3929) -> (90.3929, 53.0309) centre (90.3929, 40.3929) ccw
  line L27 (-30.3929, 51.1619) -> (90.3929, 51.1619)
  arc A12 (90.3929, -41.1619) -> (101.1619, -30.3929) centre (90.3929, -30.3929) ccw
  arc A13 (90.3929, -43.0309) -> (103.0309, -30.3929) centre (90.3929, -30.3929) ccw
  arc A14 (-41.1619, -30.3929) -> (-30.3929, -41.1619) centre (-30.3929, -30.3929) ccw
  arc A15 (-43.0309, -30.3929) -> (-30.3929, -43.0309) centre (-30.3929, -30.3929) ccw
  point P0 (30, 5)
  point P1 (30, 5)
  point P2 (30, 5)
  dimension "d36" = 144.1928
  dimension "d37" = 94.1928
  dimension "d38" = 0.9345
  dimension "d39" = 0.9345
  dimension "d40" = 0.9345
  dimension "d41" = 0.9345
  dimension "d50" = 10.769
  dimension "d51" = 12.638
  constraint midpoint L4 L8.start
  constraint midpoint L6 L8.end
  constraint midpoint L7 L9.start
  constraint midpoint L5 L9.end
  constraint horizontal L10
  constraint perpendicular L10 L11
  constraint parallel L10 L12
  constraint parallel L11 L13
  constraint coincident L14 P2
  constraint coincident L15 P2
  constraint midpoint L8 P2
  constraint horizontal L16
  constraint perpendicular L16 L17
  constraint parallel L16 L18
  constraint parallel L17 L19
  constraint coincident L20 P2
  constraint coincident L21 P2
  constraint coincident P2 P1
  constraint horizontal L22
  constraint perpendicular L22 L23
  constraint parallel L22 L27
  constraint parallel L23 L24
  constraint coincident L25 P2
  constraint coincident L26 P2
  constraint coincident L26.start L23
  constraint coincident L26.start L22
  constraint coincident L21.start L17
  constraint coincident L21.start L16
  constraint coincident L25.end L27
  constraint coincident L25.end L23
  constraint tangent A8 L27
  constraint tangent L23 A8
  constraint coincident L20.end L18
  constraint coincident L20.end L17
  constraint tangent L18 A9
  constraint tangent L17 A9
  constraint symmetric L8 A8.start A10.end
  constraint symmetric L8 L23.end L24.start
  constraint symmetric L8 A8 A10
  constraint symmetric L8 L18.start L18.end
  constraint symmetric L8 L17.end L19.start
  constraint symmetric L8 A9 A11
  constraint symmetric L9 A10.end L22.start
  constraint symmetric L9 L24.start L24.end
  constraint symmetric L9 A10 A12
  constraint symmetric L9 L18.end L16.start
  constraint symmetric L9 L19.start L19.end
  constraint symmetric L9 A11 A13
  constraint symmetric L9 A8.start L22.end
  constraint symmetric L9 L23.end L23.start
  constraint symmetric L9 A8 A14
  constraint symmetric L9 L18.start L16.end
  constraint symmetric L9 L17.end L17.start
  constraint symmetric L9 A9 A15
  constraint coincident L23.start A14.start
  constraint coincident L17.start A15.start
  constraint coincident L22.end A14.end
  constraint coincident L16.end A15.end
  measures "d36" distance of L11.end L12.end
  measures "d37" distance of L10.end L11.end
  measures "d38" distance of L13 L19
  measures "d39" distance of L13 L24
  measures "d40" distance of L10 L16
  measures "d41" distance of L10 L22
  measures "d50" radius of A8
  measures "d51" radius of A9
extrude "Extrude6" cut sketch "Sketch5" against normal blind 1.424 contours L16 L17 L18 L19 A9 A11 A13 A15
extrude "Extrude7" cut 1 faces at (50.131, -20.1369, 0) along direction (0, 0, 1) blind 0.5
sketch "Sketch6" plane through (0, 0, 0.5) normal (0, 0, -1) x (1, 0, 0)
  line L0 (90.3929, 50.4108) -> (-30.3929, 50.4108)
  arc A0 (-30.3929, 50.4108) -> (-40.4108, 40.3929) centre (-30.3929, 40.3929) ccw
  line L1 (-40.4108, 40.3929) -> (-40.4108, -30.3929)
  arc A1 (-40.4108, -30.3929) -> (-30.3929, -40.4108) centre (-30.3929, -30.3929) ccw
  line L2 (-30.3929, -40.4108) -> (90.3929, -40.4108)
  arc A2 (90.3929, -40.4108) -> (100.4108, -30.3929) centre (90.3929, -30.3929) ccw
  line L3 (100.4108, -30.3929) -> (100.4108, 40.3929)
  arc A3 (100.4108, 40.3929) -> (90.3929, 50.4108) centre (90.3929, 40.3929) ccw
  line L4 (30, 50.4108) -> (30, -40.4108) construction
  line L5 (-40.4108, 5) -> (100.4108, 5) construction
  line L6 (87.5, -35) -> (-27.5, -35)
  line L7 (-27.5, -35) -> (-27.5, 45)
  line L8 (-27.5, 45) -> (87.5, 45)
  line L9 (87.5, 45) -> (87.5, -35)
  line L10 (87.5, -35) -> (-27.5, 45) construction
  line L11 (-27.5, -35) -> (87.5, 45) construction
  point P0 (30, 5)
  dimension "d58" = 115
  dimension "d59" = 80
  constraint midpoint L0 L4.start
  constraint midpoint L2 L4.end
  constraint midpoint L1 L5.start
  constraint midpoint L3 L5.end
  constraint horizontal L6
  constraint perpendicular L6 L7
  constraint parallel L6 L8
  constraint parallel L7 L9
  constraint coincident L10 P0
  constraint coincident L11 P0
  constraint midpoint L5 P0
  measures "d58" distance of L7.end L8.end
  measures "d59" distance of L6.end L7.end
extrude "Extrude8" cut sketch "Sketch6" against normal blind 1.1 contours L6 L7 L8 L9
sketch "Sketch7" plane through (0, 0, 1.6) normal (0, 0, -1) x (1, 0, 0)
  line L0 (87.5, 45) -> (-27.5, 45)
  line L1 (-27.5, 45) -> (-27.5, -35)
  line L2 (-27.5, -35) -> (87.5, -35)
  line L3 (87.5, -35) -> (87.5, 45)
  line L4 (30, 45) -> (30, -35) construction
  line L5 (87.5, 5) -> (-27.5, 5) construction
  line L6 (85, -32.5) -> (-25, -32.5)
  line L7 (-25, -32.5) -> (-25, 42.5)
  line L8 (-25, 42.5) -> (85, 42.5)
  line L9 (85, 42.5) -> (85, -32.5)
  line L10 (85, -32.5) -> (-25, 42.5) construction
  line L11 (-25, -32.5) -> (85, 42.5) construction
  point P0 (30, 5)
  dimension "d62" = 110
  dimension "d65" = 75
  constraint midpoint L0 L4.start
  constraint midpoint L2 L4.end
  constraint midpoint L3 L5.start
  constraint midpoint L1 L5.end
  constraint horizontal L6
  constraint perpendicular L6 L7
  constraint parallel L6 L8
  constraint parallel L7 L9
  constraint coincident L10 P0
  constraint coincident L11 P0
  constraint midpoint L4 P0
  measures "d62" distance of L7.end L8.end
  measures "d65" distance of L6.end L7.end
extrude "Extrude9" cut sketch "Sketch7" against normal blind 8.4 contours L6 L7 L8 L9
equation "ORingDiameter = 1.78 mm" comment "Diamter of the O ring"
equation "ORingInnerDiameter = 150 mm" comment "Inner diamter of the o ring bore"
equation "d25 = ( ORingPerimeter - 100 mm ) / 4 + 50 mm"
equation "ORingPerimeter = 2 * 3.1412 * ( ( ORingInnerDiameter / 2 ) + ORingDiameter / 2 )"
equation "d27 = ( ORingPerimeter - 100 mm ) / 4"
equation "d28 = ( ( ORingDiameter * 1.05 ) / 2 ) + 0.5 mm"
equation "d29 = ( ( ORingDiameter * 1.05 ) / 2 ) + 0.5 mm"
equation "d30 = ( ( ORingDiameter * 1.05 ) / 2 ) + 0.5 mm"
equation "d31 = ( ( ORingDiameter * 1.05 ) / 2 ) + 0.5 mm"
equation "d32 = ORingDiameter * 0.8"
equation "d36 = ( ORingPerimeter - 100 mm ) / 4 + 50 mm"
equation "d37 = ( ORingPerimeter - 100 mm ) / 4"
equation "d38 = ( ORingDiameter * 1.05 ) / 2"
equation "d39 = ( ORingDiameter * 1.05 ) / 2"
equation "d40 = ( ORingDiameter * 1.05 ) / 2"
equation "d41 = ( ORingDiameter * 1.05 ) / 2"
equation "d44 = ( ORingDiameter ) * 6 + ORingDiameter * 0.05 - 0.5 mm"
equation "d45 = ( ORingDiameter ) * 6 + ( ORingDiameter * 1.1 ) + 0.5 mm"
equation "d50 = ( ORingDiameter ) * 6 + ORingDiameter * 0.05 - 0.0 mm"
equation "d51 = ( ORingDiameter ) * 6 + ORingDiameter * 1.1 + 0 mm"
equation "d52 = -( ORingDiameter * 0.8 )"
equation "PanelWidth = 80 mm"
equation "PanelLength = 115 mm"
equation "d58 = PanelLength"
equation "d59 = PanelWidth"
equation "d62 = PanelLength - 5 mm"
equation "d65 = PanelWidth - 5 mm"
